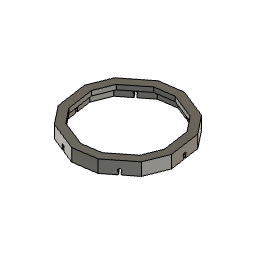
CrossSection v2 (Autodesk Fusion 360 design; units mm, degrees)
Autodesk Fusion 360 part; units mm, degrees
sketch "Sketch1" plane through (0, 0, 0) normal (0, 0, 1) x (1, 0, 0)
  line L0 (-12.2461, -1.8602) -> (-7.8071, 9.2886)
  line L1 (-7.8071, 9.2886) -> (4.0675, 11.0187)
  line L2 (4.0675, 11.0187) -> (11.5031, 1.6)
  line L3 (11.5031, 1.6) -> (7.0641, -9.5488)
  line L4 (7.0641, -9.5488) -> (-4.8105, -11.2789)
  line L5 (-4.8105, -11.2789) -> (-12.2461, -1.8602)
  line L6 (-4.8105, -11.2789) -> (7.0641, -9.5488)
  line L7 (7.0641, -9.5488) -> (9.515, -26.3712)
  line L8 (9.515, -26.3712) -> (-2.3596, -28.1013)
  line L9 (-2.3596, -28.1013) -> (-4.8105, -11.2789)
  line L10 (7.0641, -9.5488) -> (11.5031, 1.6)
  line L11 (11.5031, 1.6) -> (27.2972, -4.6887)
  line L12 (27.2972, -4.6887) -> (22.8582, -15.8374)
  line L13 (22.8582, -15.8374) -> (7.0641, -9.5488)
  line L14 (11.5031, 1.6) -> (4.0675, 11.0187)
  line L15 (4.0675, 11.0187) -> (17.4107, 21.5524)
  line L16 (17.4107, 21.5524) -> (24.8463, 12.1337)
  line L17 (24.8463, 12.1337) -> (11.5031, 1.6)
  line L18 (4.0675, 11.0187) -> (-7.8071, 9.2886)
  line L19 (-7.8071, 9.2886) -> (-10.258, 26.111)
  line L20 (-10.258, 26.111) -> (1.6166, 27.841)
  line L21 (1.6166, 27.841) -> (4.0675, 11.0187)
  line L22 (-7.8071, 9.2886) -> (-12.2461, -1.8602)
  line L23 (-12.2461, -1.8602) -> (-28.0402, 4.4284)
  line L24 (-28.0402, 4.4284) -> (-23.6012, 15.5772)
  line L25 (-23.6012, 15.5772) -> (-7.8071, 9.2886)
  line L26 (-12.2461, -1.8602) -> (-4.8105, -11.2789)
  line L27 (-4.8105, -11.2789) -> (-18.1537, -21.8127)
  line L28 (-18.1537, -21.8127) -> (-25.5893, -12.394)
  line L29 (-25.5893, -12.394) -> (-12.2461, -1.8602)
  line L30 (-28.0402, 4.4284) -> (-25.5893, -12.394)
  line L31 (-18.1537, -21.8127) -> (-2.3596, -28.1013)
  line L32 (9.515, -26.3712) -> (22.8582, -15.8374)
  line L33 (27.2972, -4.6887) -> (24.8463, 12.1337)
  line L34 (17.4107, 21.5524) -> (1.6166, 27.841)
  line L35 (-10.258, 26.111) -> (-23.6012, 15.5772)
  line L36 (-33.1811, 5.0333) -> (-27.7509, 18.6715)
  line L37 (-12.3047, 30.8656) -> (-27.7509, 18.6715)
  line L38 (-12.3047, 30.8656) -> (2.2215, 32.982)
  line L39 (20.505, 25.7021) -> (2.2215, 32.982)
  line L40 (20.505, 25.7021) -> (29.6009, 14.1803)
  line L41 (32.4381, -5.2936) -> (29.6009, 14.1803)
  line L42 (32.4381, -5.2936) -> (27.0079, -18.9317)
  line L43 (11.5616, -31.1258) -> (27.0079, -18.9317)
  line L44 (11.5616, -31.1258) -> (-2.9645, -33.2422)
  line L45 (-21.248, -25.9624) -> (-2.9645, -33.2422)
  line L46 (-21.248, -25.9624) -> (-30.3439, -14.4406)
  line L47 (-33.1811, 5.0333) -> (-30.3439, -14.4406)
  dimension "d1" = 12
  dimension "d2" = 12
  dimension "d3" = 12
  dimension "d4" = 12
  dimension "d5" = 12
  dimension "d6" = 12
  dimension "d7" = 120
  dimension "d8" = 120
  dimension "d9" = 120
  dimension "d10" = 17
  dimension "d11" = 17
  dimension "d12" = 17
  dimension "d13" = 17
  dimension "d14" = 17
  dimension "d15" = 17
  dimension "d16" = -5
  constraint perpendicular L6 L7
  constraint parallel L6 L8
  constraint parallel L7 L9
  constraint perpendicular L10 L11
  constraint parallel L10 L12
  constraint parallel L11 L13
  constraint perpendicular L14 L15
  constraint parallel L14 L16
  constraint parallel L15 L17
  constraint perpendicular L18 L19
  constraint parallel L18 L20
  constraint parallel L19 L21
  constraint perpendicular L22 L23
  constraint parallel L22 L24
  constraint parallel L23 L25
  constraint perpendicular L26 L27
  constraint parallel L26 L28
  constraint parallel L27 L29
  measures "d1" distance of L3.end L4.end
  measures "d2" distance of L0.start L4.end
  measures "d3" distance of L2.end L3.end
  measures "d4" distance of L0.end L1.end
  measures "d5" distance of L0.start L0.end
  measures "d6" distance of L1.end L2.end
  measures "d7" angle of L0 L1
  measures "d8" angle of L0 L5
  measures "d9" angle of L3 L4
  measures "d10" distance of L4.end L27.end
  measures "d11" distance of L4.end L8.end
  measures "d12" distance of L3.end L12.end
  measures "d13" distance of L2.end L16.end
  measures "d14" distance of L1.end L20.end
  measures "d15" distance of L0.end L24.end
extrude "Extrude1" add sketch "Sketch1" along normal blind 3
sketch "Sketch2" plane through (0, 0, 0) normal (0, 0, -1) x (1, 0, 0)
  line L0 (17.4107, -21.5524) -> (1.6166, -27.841)
  line L1 (1.6166, -27.841) -> (-10.258, -26.111)
  line L2 (-10.258, -26.111) -> (-23.6012, -15.5772)
  line L3 (-23.6012, -15.5772) -> (-28.0402, -4.4284)
  line L4 (-28.0402, -4.4284) -> (-25.5893, 12.394)
  line L5 (-25.5893, 12.394) -> (-18.1537, 21.8127)
  line L6 (-18.1537, 21.8127) -> (-2.3596, 28.1013)
  line L7 (-2.3596, 28.1013) -> (9.515, 26.3712)
  line L8 (9.515, 26.3712) -> (22.8582, 15.8374)
  line L9 (22.8582, 15.8374) -> (27.2972, 4.6887)
  line L10 (27.2972, 4.6887) -> (24.8463, -12.1337)
  line L11 (24.8463, -12.1337) -> (17.4107, -21.5524)
  line L12 (-27.7509, -18.6715) -> (-12.3047, -30.8656)
  line L13 (-12.3047, -30.8656) -> (2.2215, -32.982)
  line L14 (2.2215, -32.982) -> (20.505, -25.7021)
  line L15 (20.505, -25.7021) -> (29.6009, -14.1803)
  line L16 (29.6009, -14.1803) -> (32.4381, 5.2936)
  line L17 (32.4381, 5.2936) -> (27.0079, 18.9317)
  line L18 (27.0079, 18.9317) -> (11.5616, 31.1258)
  line L19 (11.5616, 31.1258) -> (-2.9645, 33.2422)
  line L20 (-2.9645, 33.2422) -> (-21.248, 25.9624)
  line L21 (-21.248, 25.9624) -> (-30.3439, 14.4406)
  line L22 (-30.3439, 14.4406) -> (-33.1811, -5.0333)
  line L23 (-33.1811, -5.0333) -> (-27.7509, -18.6715)
  line L24 (-30.3439, 14.4406) -> (-33.1811, -5.0333)
  line L25 (-30.2125, -5.4658) -> (-27.3752, 14.0081)
  line L26 (-10.4458, -28.5109) -> (-25.892, -16.3168)
  line L27 (-27.7509, -18.6715) -> (-12.3047, -30.8656)
  line L28 (19.3952, -22.915) -> (1.1117, -30.1948)
  line L29 (2.2215, -32.982) -> (20.505, -25.7021)
  line L30 (29.4695, 5.7261) -> (26.6322, -13.7478)
  line L31 (29.6009, -14.1803) -> (32.4381, 5.2936)
  line L32 (9.7027, 28.7711) -> (25.149, 16.5771)
  line L33 (27.0079, 18.9317) -> (11.5616, 31.1258)
  line L34 (-20.1382, 23.1752) -> (-1.8547, 30.455)
  line L35 (-2.9645, 33.2422) -> (-21.248, 25.9624)
  line L36 (-20.1382, 23.1752) -> (-27.3752, 14.0081)
  line L37 (-30.2125, -5.4658) -> (-25.892, -16.3168)
  line L38 (-10.4458, -28.5109) -> (1.1117, -30.1948)
  line L39 (19.3952, -22.915) -> (26.6322, -13.7478)
  line L40 (29.4695, 5.7261) -> (25.149, 16.5771)
  line L41 (9.7027, 28.7711) -> (-1.8547, 30.455)
  line L42 (-30.3439, 14.4406) -> (-21.248, 25.9624)
  line L43 (-2.9645, 33.2422) -> (11.5616, 31.1258)
  line L44 (27.0079, 18.9317) -> (32.4381, 5.2936)
  line L45 (29.4695, -14.3468) -> (20.505, -25.7021)
  line L46 (2.2215, -32.982) -> (-12.3047, -30.8656)
  line L47 (-27.7509, -18.6715) -> (-33.1811, -5.0333)
  dimension "d20" = 2
  constraint parallel L24 L25
  constraint coincident L22.end L23.start
  constraint parallel L22 L24
  constraint coincident L21.end L22.start
  constraint parallel L36 L39
  constraint parallel L37 L40
  constraint parallel L38 L41
  constraint parallel L21 L42
  constraint parallel L19 L43
  constraint parallel L17 L44
  constraint coincident L15 L45.start
  constraint parallel L15 L45
  constraint parallel L13 L46
  constraint parallel L23 L47
  measures "d20" distance of L4 L25
extrude "Extrude2" add sketch "Sketch2" along normal blind 5 contours L12 L13 L14 L15 L16 L17 L18 L19 L20 L21 L22 L23 L24 L27 L29 L31 L33 L35 L42 L43 L44 L45 L46 L47
sketch "Sketch3" plane through (17.718, -22.4435, 0) normal (-0.619633, 0.784891, 0) x (-0.784891, -0.619633, 0)
  line L0 (10.212, 0) -> (-9.4675, 0)
  line L1 (-9.4675, 0) -> (-9.4675, -5)
  line L2 (-9.4675, -5) -> (10.212, -5)
  line L3 (10.212, -5) -> (10.212, 0)
  line L4 (1.005, -5) -> (-0.2606, -5)
  line L5 (-0.2606, -5) -> (-0.2606, -3.2743)
  line L6 (1.005, -3.2743) -> (1.005, -5)
  arc A0 (1.005, -3.2743) -> (-0.2606, -3.2743) centre (0.3722, -2.5) ccw
  point P0 (0.3722, -2.5)
  dimension "d25" = 2
  constraint horizontal L4
  constraint perpendicular L4 L5
  constraint coincident L2 L4.start
  constraint coincident P0 A0.centre
  measures "d25" diameter of A0
extrude "Extrude3" cut sketch "Sketch3" against normal blind 7 contours L2 L4 L5 L6 A0
pattern_circular "C-Pattern1" count 6 over 360 about axis through (-0.3715, -0.1301, 1) along (0, 0, -1) of "Extrude3"
